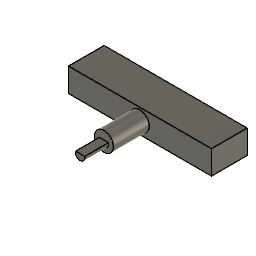
attache_roue_4mm_diametres (Autodesk Fusion 360 design; units mm, degrees)
part number: 2026-05-27-08-20-16-323
Autodesk Fusion 360 part; units mm, degrees
sketch "Esquisse1" plane through (0, 0, 0) normal (0, 1, 0) x (1, 0, 0)
  circle A0 centre (0, 0) radius 4
  dimension "d1" = 8
  constraint coincident A0.centre origin
  measures "d1" diameter of A0
extrude "Extrusion1" add sketch "Esquisse1" along normal blind 15
sketch "Esquisse2" plane through (0, 15, 0) normal (0, 1, 0) x (-1, 0, 0)
  circle A0 centre (0, 0) radius 4
  line L0 (-30.089, 4.9107) -> (29.911, 4.9107)
  line L1 (29.911, 4.9107) -> (29.911, -5.0893)
  line L2 (29.911, -5.0893) -> (-30.089, -5.0893)
  line L3 (-30.089, -5.0893) -> (-30.089, 4.9107)
  point P0 (-0.089, -5.0893)
  dimension "d12" = 60
  dimension "d13" = 10
  constraint horizontal L0
  constraint vertical L1
  constraint horizontal L2
  constraint vertical L3
  constraint midpoint L2 P0
  measures "d12" distance of L0.start L0.end
  measures "d13" distance of L0.end L1.end
extrude "Extrusion2" add sketch "Esquisse2" along normal blind 15 contours A0 | L0 L1 L2 L3
sketch "Esquisse5" plane through (0, 0, 0) normal (0, -1, 0) x (1, 0, 0)
  circle A0 centre (0, 0) radius 4
  circle A1 centre (0, 0) radius 2
  dimension "d14" = 4
  constraint concentric A0 A1
  measures "d14" diameter of A1
extrude "Extrusion4" add sketch "Esquisse5" along normal blind 10 contours A1
sketch "Esquisse7" plane through (0, 0, 0) normal (1, 0, 0) x (0, 1, 0)
  line L0 (-10, 2) -> (0, 2)
  line L1 (0, 2) -> (0, 0.5)
  line L2 (0, 0.5) -> (-10, 0.5)
  line L3 (-10, 0.5) -> (-10, 2)
  dimension "d19" = 10
  dimension "d20" = 1.5
  constraint horizontal L0
  constraint vertical L1
  constraint horizontal L2
  constraint vertical L3
  measures "d19" distance of L0.start L0.end
  measures "d20" distance of L0.start L2.end
extrude "Extrusion5" cut sketch "Esquisse7" along normal blind 3.5 and the other way blind 3
